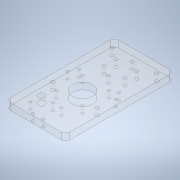
# Autodesk Inventor part: Gripper_Base_new
Saved by Autodesk Inventor 2022 (Build 260153000, 153)
## iProperties
Created: 2021-04-16
Part Number: Gripper_Base_new
Material: PET Plastic
Document SubType Name: Modeling
Designer: domin
Density: 1.541 g/cm^3
Appearance: Polycarbonate - Clear
Mass: 94.2221 g
Surface Area: 209.833 cm^2
Volume: 61.1435 cm^3
Author: domin
Autodesk Inventor part; units mm, degrees
ref_plane "YZ Plane" through (0, 0, 0) normal (1, 0, 0) x (0, 1, 0)
ref_plane "XZ Plane" through (0, 0, 0) normal (0, 1, 0) x (-1, 0, 0)
ref_plane "XY Plane" through (0, 0, 0) normal (0, 0, 1) x (1, 0, 0)
sketch "Sketch1" plane through (0, 0, 0) normal (0, 1, 0) x (-1, 0, 0)
  line L0 (35, 99.5) -> (-35, 99.5)
  line L1 (-35, 99.5) -> (-35, -27.999)
  line L2 (-35, -27.999) -> (35, -27.999)
  line L3 (35, -27.999) -> (35, 99.5)
  line L4 (26.1865, 53.5) -> (-26.1865, 53.5) construction
  line L5 (-26.1865, 53.5) -> (-26.1865, -16.5) construction
  line L6 (-26.1865, -16.5) -> (26.1865, -16.5) construction
  line L7 (26.1865, -16.5) -> (26.1865, 53.5) construction
  circle A0 centre (26.1865, 53.5) radius 4 construction
  circle A1 centre (-26.1865, 53.5) radius 4 construction
  circle A2 centre (-26.1865, -16.5) radius 4 construction
  circle A3 centre (26.1865, -16.5) radius 4 construction
  circle A4 centre (0, 40) radius 15 construction
  line L8 (20.5, 20.5) -> (-20.5, 20.5) construction
  line L9 (-20.5, 20.5) -> (-20.5, -20.5) construction
  line L10 (-20.5, -20.5) -> (20.5, -20.5) construction
  line L11 (20.5, -20.5) -> (20.5, 20.5) construction
  point P0 (0, 0)
  dimension "d57" = 127.499
  dimension "d58" = 70
  dimension "d59" = 8
  dimension "d60" = 8
  dimension "d61" = 8
  dimension "d62" = 8
  dimension "d63" = 70
  dimension "d64" = 52.373
  dimension "d66" = 8.8135
  dimension "d67" = 46
  dimension "d70" = 30
  dimension "d71" = 41
  dimension "d72" = 41
  dimension "d73" = 20.5
  dimension "d74" = 20.5
  dimension "d75" = 40
  dimension "d76" = 35
  dimension "d210" = 16.5
  constraints: 24 end point, 6 parallel, 5 centre point, 4 coincident, 3 horizontal, 3 perpendicular
  measures "d57" distance between parallel lines of L2 L0
  measures "d58" distance of L0.start L0.end
  measures "d59" diameter of A0
  measures "d60" diameter of A1
  measures "d61" diameter of A2
  measures "d62" diameter of A3
  measures "d63" distance of L5.end L4.end
  measures "d64" distance of L4.end L4.start
  measures "d66" horizontal distance of L4.start L0.start
  measures "d67" vertical distance of L0.end L4.end
  measures "d70" diameter of A4
  measures "d71" distance of L8.end L9.end
  measures "d72" distance between parallel lines of L9 L11
  measures "d73" distance from line of point (0, 0) L8
  measures "d74" horizontal distance of point (0, 0) L10.end
  measures "d75" distance of point (0, 0) A4.centre
  measures "d76" distance from line of L3 point (0, 0)
  measures "d210" vertical distance of L6.end point (0, 0)
extrude "Extrusion1" add sketch "Sketch1" along normal blind 8
sketch "Sketch7" plane through (0, 8, 0) normal (0, 1, 0) x (1, 0, 0)
  circle A0 centre (0, -44.501) radius 12
  line L0 (35, 27.999) -> (-35, 27.999) projected
  line L1 (-35, 27.999) -> (-35, -99.5) projected
  dimension "d77" = 24
  dimension "d205" = 72.5
  dimension "d206" = 35
  constraints: 1 centre point, 1 coincident
  measures "d77" diameter of A0
  measures "d205" distance from line of L0 point (0, -44.501)
  measures "d206" distance from line of point (0, -44.501) L1
hole "MotormainHole5" at (0, 8, 44.501) direction (0, -1, 0) diameter 24 end through all
sketch "Sketch8" plane through (0, 8, 0) normal (0, 1, 0) x (1, 0, 0)
  line L0 (15.5, -60.001) -> (-15.5, -60.001) construction
  line L1 (-15.5, -60.001) -> (-15.5, -29.001) construction
  line L2 (-15.5, -29.001) -> (15.5, -29.001) construction
  line L3 (15.5, -29.001) -> (15.5, -60.001) construction
  circle A0 centre (15.5, -60.001) radius 1.5
  circle A1 centre (-15.5, -60.001) radius 1.5
  circle A2 centre (-15.5, -29.001) radius 1.5
  circle A3 centre (15.5, -29.001) radius 1.5
  circle A4 centre (0, -44.501) radius 12 projected
  point P0 (0, 0)
  dimension "d85" = 3
  dimension "d86" = 31
  dimension "d87" = 31
  dimension "d88" = 15.5
  dimension "d215" = 15.5
  constraints: 8 end point, 4 centre point, 4 coincident, 3 equal radius, 2 parallel, 1 horizontal, 1 perpendicular
  measures "d85" diameter of A0
  measures "d86" distance of L0.start L0.end
  measures "d87" distance of L2.end L0.start
  measures "d88" horizontal distance of L0.start point (0, 0)
  measures "d215" horizontal distance of A4.centre L0.start
hole "MotorHole6" at (15.5, 8, 60.001) at (-15.5, 8, 60.001) at (-15.5, 8, 29.001) at (15.5, 8, 29.001) direction (0, -1, 0) diameter 3 end through all
sketch "Sketch9" plane through (0, 0, 0) normal (0, -1, 0) x (1, 0, 0)
  circle A0 centre (-5, 74.501) radius 1.5
  circle A1 centre (5, 74.501) radius 1.5
  line L0 (-35, -27.999) -> (-35, 99.5) projected
  line L1 (35, 99.5) -> (35, -27.999) projected
  circle A2 centre (0, 44.501) radius 12 projected
  point P0 (0, 0)
  dimension "d97" = 3
  dimension "d186" = 30
  dimension "d187" = 30
  dimension "d207" = 30
  constraints: 2 centre point, 1 equal radius, 1 horizontal alignment
  measures "d97" diameter of A0
  measures "d186" distance from line of L1 A1.centre
  measures "d187" distance from line of L0 A0.centre
  measures "d207" vertical distance of A2.centre A1.centre
hole "GrippersupportHole7" at (-5, 0, 74.501) at (5, 0, 74.501) direction (0, 1, 0) diameter 3 end through all
sketch "Sketch10" plane through (0, 8, 0) normal (0, 1, 0) x (1, 0, 0)
  line L0 (26.1865, -53.5) -> (-26.1865, -53.5) construction
  line L1 (-26.1865, -53.5) -> (-26.1865, 16.5) construction
  line L2 (-26.1865, 16.5) -> (26.1865, 16.5) construction
  line L3 (26.1865, 16.5) -> (26.1865, -53.5) construction
  circle A0 centre (26.1865, -53.5) radius 2.15
  circle A1 centre (-26.1865, -53.5) radius 2.15
  circle A2 centre (-26.1865, 16.5) radius 2.15
  circle A3 centre (26.1865, 16.5) radius 2.15
  line L4 (35, -99.5) -> (35, 27.999) projected
  line L5 (-35, -99.5) -> (35, -99.5) projected
  point P0 (0, 0)
  dimension "d111" = 4.3
  dimension "d112" = 8.8135
  dimension "d113" = 52.373
  dimension "d114" = 46
  dimension "d115" = 70
  constraints: 8 end point, 4 centre point, 4 coincident, 3 equal radius, 2 parallel, 1 horizontal, 1 perpendicular
  measures "d111" diameter of A0
  measures "d112" distance from line of L4 L0.start
  measures "d113" distance of L0.end L0.start
  measures "d114" distance between parallel lines of L5 L0
  measures "d115" distance of L1.end L0.end
hole "supportHole8" at (26.1865, 8, 53.5) at (-26.1865, 8, 53.5) at (26.1865, 8, -16.5) at (-26.1865, 8, -16.5) direction (0, -1, 0) diameter 4.3 end through all
sketch "Sketch11" plane through (0, 0, 0) normal (0, -1, 0) x (1, 0, 0)
  circle A0 centre (0, 0) radius 14 construction
  circle A1 centre (-26.1865, 53.5) radius 2.15 projected
  circle A2 centre (26.1865, 53.5) radius 2.15 projected
  circle A3 centre (0, 14) radius 2
  circle A4 centre (-12.1244, 7) radius 2
  circle A5 centre (-12.1244, -7) radius 2
  circle A6 centre (0, -14) radius 2
  line L0 (35, -27.999) -> (-35, -27.999) projected
  circle A7 centre (-26.1865, -16.5) radius 2.15 projected
  circle A8 centre (26.1865, -16.5) radius 2.15 projected
  circle A9 centre (12.1244, -7) radius 2
  circle A10 centre (12.1244, 7) radius 2
  point P0 (0, 0)
  dimension "d125" = 28
  dimension "d126" = 4
  dimension "d129" = 360
  dimension "d213" = 16.5
  dimension "d214" = 0
  constraints: 6 centre point, 2 vertical alignment, 15 other
  measures "d126" diameter of A3
  measures "d213" vertical distance of A7.centre point (0, 0)
  measures "d214" distance of point (0, 0) point (0, 0)
hole "ScrewHole9" at (0, 0, 14) at (0, 0, -14) at (-12.1244, 0, -7) at (-12.1244, 0, 7) direction (0, 1, 0) diameter 4 end through all
fillet "MainFillet1" radius 5 4 edges at (-35, 4, 99.5) (35, 4, 99.5) (35, 4, -27.999) (-35, 4, -27.999)
sketch "Sketch12" plane through (0, 8, 0) normal (0, 1, 0) x (1, 0, 0)
  circle A0 centre (-19, -74) radius 4
  point P0 (0, 0)
  dimension "d139" = 8
  dimension "d140" = 19
  dimension "d141" = 74
  constraints: 1 centre point
  measures "d139" diameter of A0
  measures "d140" horizontal distance of A0.centre point (0, 0)
  measures "d141" vertical distance of point (0, 0) A0.centre
hole "Wirehole" at (-19, 8, 74) direction (0, -1, 0) diameter 8 end through all
sketch "Sketch13" plane through (0, 0, 0) normal (0, -1, 0) x (1, 0, 0)
  circle A0 centre (-19, 87) radius 1.5
  circle A1 centre (-19, 74) radius 4 projected
  line L0 (-19, 74) -> (-19, 90.0353) construction
  line L1 (-19, 74) -> (-19, 87) construction
  point P0 (0, 0)
  dimension "d149" = 3
  dimension "d211" = 13
  dimension "d212" = 0
  constraints: 4 end point, 1 centre point, 1 vertical
  measures "d149" diameter of A0
  measures "d211" distance of L0.start L1.end
  measures "d212" distance between parallel lines of L0 L1
hole "Hole11" at (-19, 0, 87) direction (0, 1, 0) diameter 3 end through all
sketch "Sketch16" plane through (0, 8, 0) normal (0, 1, 0) x (1, 0, 0)
  circle A0 centre (-6, -97) radius 1.6
  circle A1 centre (6, -97) radius 1.6
  line L0 (-30, -99.5) -> (30, -99.5) projected
  circle A2 centre (-26.1865, -53.5) radius 2.15 projected
  point P0 (0, 0)
  point P1 (-20, -99.5)
  dimension "d173" = 3.2
  dimension "d174" = 12
  dimension "d175" = 6
  dimension "d216" = 43.5
  constraints: 2 centre point, 1 equal radius, 1 horizontal alignment
  measures "d173" diameter of A0
  measures "d174" distance of A0.centre A1.centre
  measures "d175" horizontal distance of point (0, 0) A0.centre
  measures "d216" vertical distance of A2.centre A0.centre
hole "chainHole13" at (-6, 8, 97) at (6, 8, 97) direction (0, -1, 0) diameter 3.2 end through all
sketch "Sketch17" plane through (0, 8, 0) normal (0, 1, 0) x (1, 0, 0)
  circle A0 centre (-5, -74.501) radius 1.5
  circle A1 centre (5, -74.501) radius 1.5
  circle A2 centre (-5, -74.501) radius 1.5 projected
  circle A3 centre (5, -74.501) radius 1.5 projected
  circle A4 centre (28.4808, -33.8311) radius 1.5
  circle A5 centre (23.4808, -25.1709) radius 1.5
  circle A6 centre (-23.4808, -25.1709) radius 1.5
  circle A7 centre (-28.4808, -33.8311) radius 1.5
  circle A8 centre (0, -44.501) radius 12 projected
  dimension "d188" = 0
  dimension "d189" = 0
  dimension "d190" = 3
  dimension "d193" = 360
  dimension "d208" = 0
  dimension "d209" = 0
  constraints: 6 centre point, 2 coincident, 1 equal radius, 13 other
  measures "d188" distance of A2.centre A0.centre
  measures "d189" distance of A3.centre A1.centre
  measures "d190" diameter of A0
  measures "d208" distance of point (0, -44.501) A8.centre
  measures "d209" distance of A8.centre point (0, -44.501)
hole "Grippersupport2Hole14" at (23.4808, 8, 25.1709) at (28.4808, 8, 33.8311) at (-28.4808, 8, 33.8311) at (-23.4808, 8, 25.1709) direction (0, -1, 0) diameter 3 end through all
sketch "Sketch18" plane through (0, 8, 0) normal (0, 1, 0) x (1, 0, 0)
  circle A0 centre (0, 0) radius 14
  line L0 (0, 0) -> (16.8596, -9.7339)
  line L1 (0, 0) -> (20.1281, 11.6209)
  line L2 (0, 0) -> (0, -20)
  point P0 (12.1244, 7)
  point P1 (12.1244, -7)
  dimension "d217" = 28
  dimension "d218" = 20
  dimension "d219" = 60
  dimension "d220" = 120
  constraints: 6 end point, 2 point on circle, 2 point on line, 1 centre point, 1 coincident, 1 vertical
  measures "d217" diameter of A0
  measures "d218" distance of L0.start L2.end
  measures "d219" angle of L2 L0
  measures "d220" angle of L2 L1
hole "Hole15" at (12.1244, 8, 7) at (12.1244, 8, -7) direction (0, -1, 0) diameter 4 end through all
equation "\"d66\" = -0.5 * d64 + 0.5 * d58"
equation "\"d73\" = 0.5 * d71"
equation "\"d74\" = 0.5 * d72"
equation "\"d76\" = 0.5 * d58"
equation "\"d78\" = d77"
equation "\"d88\" = 0.5 * d86"
equation "\"d90\" = d85"
equation "\"d101\" = d97"
equation "\"d112\" = d66"
equation "\"d113\" = d64"
equation "\"d114\" = d67"
equation "\"d115\" = d63"
equation "\"d116\" = d111"
equation "\"d142\" = d139"
equation "\"d175\" = 0.5 * d174"
equation "\"d177\" = d173"
equation "\"d195\" = d190"
body "Solid1"
